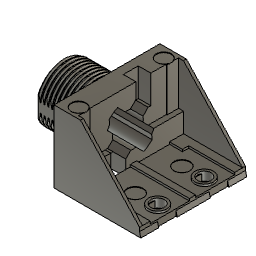
Cherry Pushbutton Base (Autodesk Fusion 360 design; units mm, degrees)
Autodesk Fusion 360 part; units mm, degrees
sketch "Sketch1" plane through (0, 0, 0) normal (0, 1, 0) x (1, 0, 0)
  line L0 (0, 0) -> (0, -14.6844)
  line L1 (0, -14.6844) -> (5.4102, -14.6844)
  line L2 (5.4102, -14.6844) -> (17.4625, -1.778)
  line L3 (17.4625, -1.778) -> (17.4625, 0)
  line L4 (17.4625, 0) -> (0, 0)
  dimension "d12" = 1.778
  dimension "d14" = 17.4625
  dimension "d16" = 14.6844
  dimension "d18" = 5.4102
  constraint coincident L0.start L4.end
  constraint vertical L0
  constraint perpendicular L0 L1
  constraint perpendicular L1 L3
  constraint perpendicular L0 L4
  measures "d12" distance of L2.end L3.end
  measures "d14" distance of L3.end L0.start
  measures "d16" distance of L0.start L0.end
  measures "d18" distance of L0.end L1.end
extrude "Extrude1" add sketch "Sketch1" along normal mid plane 21.6154
ref_plane "WorkPlane1" through (17.4625, 0, 1.778) normal (0, 0, 1) x (0, 1, 0)
sketch "Sketch3" plane through (0, 0, 1.778) normal (0, 0, 1) x (1, 0, 0)
  line L0 (5.4102, -10.8077) -> (5.4102, 10.8077)
  line L1 (17.4625, -10.8077) -> (17.4625, 10.8077)
  line L2 (17.4625, 10.2124) -> (5.4102, 10.2124)
  line L3 (5.4102, 10.2124) -> (5.4102, -10.2124)
  line L4 (5.4102, -10.2124) -> (17.4625, -10.2124)
  line L5 (17.4625, -10.2124) -> (17.4625, 10.2124)
  line L6 (0, 0) -> (5.4102, 0) construction
  dimension "d7" = 20.4248
  constraint horizontal L2
  constraint vertical L3
  constraint horizontal L4
  constraint vertical L5
  constraint coincident L0 L3.end
  constraint coincident L1 L2.start
  constraint coincident L6.start origin
  constraint midpoint L3 L6.end
  constraint horizontal L6
  measures "d7" distance of L2.start L4.end
extrude "Extrude2" cut sketch "Sketch3" along normal up to surface (12.9064 mm away)
sketch "Sketch4" plane through (0, 0, 0) normal (-1, 0, 0) x (0, -1, 0)
  line L0 (10.8077, 14.6844) -> (-10.8077, 14.6844)
  line L1 (-10.8077, 14.6844) -> (-10.8077, 0)
  line L2 (-10.8077, 0) -> (10.8077, 0)
  line L3 (10.8077, 0) -> (10.8077, 14.6844)
  line L4 (-10.8077, 0) -> (10.8077, 14.6844) construction
  circle A0 centre (0, 7.3422) radius 5.3975
  line L5 (-5.3975, 14.6844) -> (5.3975, 14.6844)
  line L6 (5.3975, 14.6844) -> (5.3975, 0)
  line L7 (5.3975, 0) -> (-5.3975, 0)
  line L8 (-5.3975, 0) -> (-5.3975, 14.6844)
  point P0 (0, 7.3422)
  dimension "d87" = 10.795
  constraint coincident L1.end L2.start
  constraint coincident L0.start L3.end
  constraint midpoint L4 P0
  constraint coincident P0 A0.centre
  constraint horizontal L5
  constraint vertical L6
  constraint horizontal L7
  constraint vertical L8
  constraint coincident L2 L6.end
  constraint coincident L0 L5.start
  constraint tangent A0 L6
  constraint tangent A0 L8
  measures "d87" diameter of A0
extrude "Extrude3" add sketch "Sketch4" along normal blind 9.1281 contours A0
sketch "Sketch5" plane through (-9.1281, 0, 0) normal (-1, 0, 0) x (0, -1, 0)
  circle A0 centre (0, 7.3422) radius 4.4323
  circle A1 centre (0, 7.3422) radius 5.3975
  dimension "d33" = 8.8646
  constraint concentric A0 A1
  measures "d33" diameter of A0
extrude "Extrude4" cut sketch "Sketch5" against normal up to surface (14.5383 mm away) contours A0
thread "Thread2" "Custom ANSI Unified Screw Threads 15/32 15/32-32 UN 2A" major diameter 11.684 minor diameter 10.9626 pitch 0.7937 angle 60 modelled right hand crest width 0.2004 on face at (-3.0427, -5.3707, 6.8048) crest through (0.1984, -5.842, 7.3422)
sketch "Sketch6" plane through (5.4102, 0, 0) normal (1, 0, 0) x (0, 1, 0)
  circle A0 centre (0, 7.3422) radius 4.4323
  line L0 (10.2124, 14.6844) -> (-10.2124, 14.6844)
  line L1 (-10.2124, 14.6844) -> (-10.2124, 1.778)
  line L2 (-10.2124, 1.778) -> (10.2124, 1.778)
  line L3 (10.2124, 1.778) -> (10.2124, 14.6844)
  circle A1 centre (0, 7.3422) radius 3.1369
  line L4 (-0.5334, 10.4334) -> (0.5334, 10.4334) construction
  line L5 (0, 14.6844) -> (0, 1.778) construction
  line L6 (0, 10.4791) -> (0, 10.4334) construction
  line L7 (0.5334, 10.4334) -> (1.5824, 11.4824)
  line L8 (-0.5334, 10.4334) -> (-1.5824, 11.4824)
  line L9 (-3.0912, 6.8088) -> (-4.1402, 5.7598)
  line L10 (-3.0912, 6.8088) -> (-3.0912, 7.8756) construction
  line L11 (-3.0912, 7.8756) -> (-4.1402, 8.9246)
  line L12 (-3.1369, 7.3422) -> (-3.0912, 7.3422) construction
  line L13 (0.5334, 4.251) -> (1.5824, 3.202)
  line L14 (0.5334, 4.251) -> (-0.5334, 4.251) construction
  line L15 (-0.5334, 4.251) -> (-1.5824, 3.202)
  line L16 (0, 4.2053) -> (0, 4.251) construction
  line L17 (3.0912, 7.8756) -> (4.1402, 8.9246)
  line L18 (3.0912, 7.8756) -> (3.0912, 6.8088) construction
  line L19 (3.0912, 6.8088) -> (4.1402, 5.7598)
  line L20 (3.1369, 7.3422) -> (3.0912, 7.3422) construction
  line L21 (1.5824, 11.4824) -> (0, 10.4334) construction
  line L22 (-1.5824, 11.4824) -> (0, 10.4334) construction
  line L23 (-4.1402, 5.7598) -> (-4.1402, 0)
  line L24 (-1.5824, 3.202) -> (-1.5824, 0)
  line L25 (10.8077, 0) -> (-10.8077, 0)
  line L26 (-10.2124, 14.6844) -> (10.2124, 14.6844)
  line L27 (10.2124, 14.6844) -> (10.2124, 5.769)
  line L28 (10.2124, 5.769) -> (-10.2124, 5.769)
  line L29 (-10.2124, 5.769) -> (-10.2124, 14.6844)
  circle A2 centre (0, 7.3422) radius 5.0927
  line L30 (-1.5824, 11.4824) -> (-2.0874, 11.9874)
  line L31 (1.5824, 3.202) -> (2.0874, 2.6969)
  line L32 (-2.0874, 11.9874) -> (-3.7985, 10.7343) construction
  line L33 (-3.7985, 10.7343) -> (-3.7214, 9.7497)
  line L34 (-3.6157, 8.4001) -> (-3.7214, 9.7497)
  line L35 (1.5824, 3.202) -> (2.0874, 2.6969)
  line L36 (2.0874, 2.6969) -> (3.7985, 3.95) construction
  line L37 (3.7985, 3.95) -> (3.7214, 4.9346)
  line L38 (3.6157, 6.2843) -> (3.7214, 4.9346)
  point P0 (4.4323, 7.3422)
  point P1 (0, 7.3422)
  point P2 (0, 10.4791)
  point P3 (0, 10.4334)
  point P4 (-3.0912, 7.3422)
  point P5 (-3.1369, 7.3422)
  point P6 (0, 4.251)
  point P7 (0, 4.2053)
  point P8 (3.0912, 7.3422)
  point P9 (3.1369, 7.3422)
  dimension "d38" = 6.2738
  dimension "d39" = 1.0668
  dimension "d41" = 360
  dimension "d72" = 8.9154
  dimension "d88" = 20.4248
  dimension "d90" = 10.1854
  dimension "d92" = 2.1209
  dimension "d94" = 360
  constraint coincident P1 A0.centre
  constraint perpendicular L3 L4
  constraint coincident L5 P2
  constraint coincident A1 P2
  constraint midpoint L4 P3
  constraint coincident P2 L6.start
  constraint coincident P3 L6.end
  constraint vertical L6
  constraint coincident A1 L4.end
  constraint coincident A0 L7.end
  constraint coincident A0 L8.end
  constraint equal L21 L22
  constraint parallel L8 L11
  constraint perpendicular L2 L23
  constraint perpendicular L2 L24
  constraint coincident L23.end L25
  constraint coincident L24.end L25
  constraint horizontal L26
  constraint vertical L27
  constraint horizontal L28
  constraint vertical L29
  constraint coincident L0.end L1.start
  constraint coincident A2 L30.end
  constraint collinear L8 L30
  constraint coincident A2 L31.end
  constraint collinear L13 L31
  constraint coincident A2 L32.end
  constraint coincident A0 L33.end
  constraint coincident L11 L34.start
  constraint midpoint L11 L34.start
  constraint collinear L33 L34
  measures "d38" diameter of A1
  measures "d39" distance of L4.start L4.end
  measures "d72" distance of L0.end L28.end
  measures "d88" distance of L27.end L28.end
  measures "d90" diameter of A2
  measures "d92" distance of L30.end L32.end
extrude "Extrude5" add sketch "Sketch6" against normal blind 7.366 contours A0 A1 L17 L19 L28 | A0 L19 L28 | A0 A1 L7 L8 | A0 A1 L13 L15 | A0 A1 L9 L11 L28 | A0 L9 L28
sketch "Sketch7" plane through (0, 0, 14.6844) normal (0, 0, 1) x (-1, 0, 0)
  line L0 (-5.4102, 10.8077) -> (-5.4102, 10.2124)
  line L1 (-5.4102, 10.2124) -> (-5.4102, -10.2124)
  line L2 (-5.4102, -10.2124) -> (-5.4102, -10.8077)
  line L3 (-5.4102, -10.8077) -> (0, -10.8077)
  line L4 (0, -10.8077) -> (0, 10.8077)
  line L5 (0, 10.8077) -> (-5.4102, 10.8077)
  line L6 (-5.4102, -1.6383) -> (-1.7018, -1.6383)
  line L7 (-1.7018, -1.6383) -> (-1.7018, -4.6863)
  line L8 (-1.7018, -4.6863) -> (-5.4102, -4.6863)
  line L9 (-5.4102, -4.6863) -> (-5.4102, -1.6383)
  line L10 (-3.556, -4.6863) -> (-3.556, -10.8077) construction
  dimension "d50" = 15.494
  dimension "d51" = 12.446
  dimension "d61" = 3.048
  dimension "d62" = 1.7018
  dimension "d64" = 6.1214
  constraint horizontal L6
  constraint vertical L7
  constraint horizontal L8
  constraint vertical L9
  constraint coincident L1 L6.start
  constraint midpoint L8 L10.start
  constraint coincident L3 L10.end
  constraint perpendicular L3 L10
  measures "d50" distance of L5 L8
  measures "d51" distance of L5 L6
  measures "d61" distance of L6.end L7.end
  measures "d62" distance of L4 L7
  measures "d64" distance of L10.start L10.end
extrude "Extrude6" cut sketch "Sketch7" against normal up to surface (5.7598 mm away) contours L1 L6 L7 L8 L9
extrude "Extrude7" cut sketch "Sketch6" against normal up to surface (3.7084 mm away) contours A0 L23 L24 A2 | L2 L23 L24 L25 | L2 L23 L24 A2
sketch "Sketch10" plane through (0, 0, 0) normal (0, 0, -1) x (1, 0, 0)
  line L0 (5.4102, 4.1402) -> (5.4102, 1.5824)
  line L1 (5.4102, 1.5824) -> (1.7018, 1.5824)
  line L2 (1.7018, 1.5824) -> (1.7018, 4.1402)
  line L3 (0, 10.8077) -> (0, -10.8077)
  line L4 (0, -10.8077) -> (17.4625, -10.8077)
  line L5 (17.4625, -10.8077) -> (17.4625, 10.8077)
  line L6 (17.4625, 10.8077) -> (0, 10.8077)
  line L7 (1.7018, 4.1402) -> (5.4102, 4.1402)
sketch "Sketch11" plane through (0, 0, 0) normal (0, 0, -1) x (1, 0, 0)
  line L0 (5.4102, 1.5824) -> (1.7018, 1.5824)
  line L1 (1.7018, 1.5824) -> (1.7018, 4.6304)
  line L2 (1.7018, 4.6304) -> (5.4102, 4.6304)
  line L3 (5.4102, 4.6304) -> (5.4102, 1.5824)
  point P0 (5.4102, 1.5824)
  point P1 (1.7018, 1.5824)
  dimension "d66" = 3.048
  constraint horizontal L0
  constraint vertical L1
  constraint horizontal L2
  constraint vertical L3
  constraint coincident P0 L0.start
  constraint coincident P1 L1
  measures "d66" distance of P0 L2.end
extrude "Extrude9" cut sketch "Sketch11" against normal up to surface (1.778 mm away)
extrude "Extrude10" cut 1 faces at (2.9379, -4.1402, 4.4325) along direction (0, -1, 0) up to surface (0.4902 mm away)
sketch "Sketch12" plane through (0, -4.95, 4.95) normal (0, 0.707107, -0.707107) x (-1, 0, 0)
  line L0 (-5.4102, 2.6287) -> (-5.4102, 1.1452)
  line L1 (-5.4102, 1.1452) -> (-1.7018, 1.1452)
  line L2 (-1.7018, 1.1452) -> (1.9558, 1.1452)
  line L3 (1.9558, 1.1452) -> (1.9558, 2.6287)
  line L4 (1.9558, 2.6287) -> (-5.4102, 2.6287)
extrude "Extrude11" cut sketch "Sketch6" against normal blind 1.143 contours A0 A1 L17 L19 L28 | A0 L28 A2 L30 | A0 L19 L28 | A0 A1 L7 L8 | L0 L1 L3 L26 L27 L28 L29 A2 | A0 A2 L30 L33 | A0 L28 A2 L33 | A0 A1 L9 L11 L28 | A0 L9 L28
sketch "Sketch13" plane through (4.2672, 0, 0) normal (1, 0, 0) x (0, 1, 0)
  line L0 (1.6383, 11.4606) -> (1.6383, 14.6844)
  line L1 (1.6383, 14.6844) -> (-10.2124, 14.6844)
  line L2 (-10.2124, 14.6844) -> (-10.2124, 5.769)
  line L3 (-10.2124, 5.769) -> (-4.1437, 5.769)
  line L4 (-4.1402, 5.7598) -> (-3.0912, 6.8088)
  arc A0 (-3.0912, 7.8756) -> (-3.0912, 6.8088) centre (0, 7.3422) ccw
  line L5 (-3.0912, 7.8756) -> (-4.1402, 8.9246)
  arc A1 (-1.5824, 11.4824) -> (-4.1402, 8.9246) centre (0, 7.3422) ccw
  line L6 (-1.5824, 11.4824) -> (-0.5334, 10.4334)
  arc A2 (0.5334, 10.4334) -> (-0.5334, 10.4334) centre (0, 7.3422) ccw
  line L7 (0.5334, 10.4334) -> (1.5824, 11.4824)
  line L8 (-10.2124, 14.6844) -> (-7.874, 14.6844)
  line L9 (-7.874, 14.6844) -> (-7.874, 5.769)
  line L10 (-7.874, 5.769) -> (-10.2124, 5.769)
  line L11 (-10.2124, 5.769) -> (-10.2124, 14.6844)
  line L12 (10.2124, 5.769) -> (-10.2124, 5.769)
  line L13 (10.2124, 14.6844) -> (10.2124, 5.769)
  line L14 (10.2124, 14.6844) -> (7.874, 14.6844)
  line L15 (7.874, 14.6844) -> (7.874, 5.769)
  line L16 (7.874, 5.769) -> (10.2124, 5.769)
  line L17 (10.2124, 5.769) -> (10.2124, 14.6844)
  arc A3 (-4.1437, 5.769) -> (-4.1402, 5.7598) centre (0, 7.3422) ccw
  arc A4 (1.6383, 11.4606) -> (1.5824, 11.4824) centre (0, 7.3422) ccw
  dimension "d76" = 2.3384
  dimension "d77" = 2.3384
  constraint horizontal L8
  constraint vertical L9
  constraint horizontal L10
  constraint vertical L11
  constraint coincident L1.end L2.start
  constraint collinear L10 L12
  constraint horizontal L14
  constraint vertical L15
  constraint horizontal L16
  constraint vertical L17
  constraint coincident L13.start L14.start
  constraint coincident L9.end L12
  constraint collinear L12 L16
  measures "d76" distance of L1.end L8.end
  measures "d77" distance of L13.start L14.end
extrude "Extrude12" add sketch "Sketch13" along normal blind 0.127 contours L1 L2 L3 L8 L9 L10 L11 L12 | L12 L13 L14 L15 L16 L17
sketch "Sketch14" plane through (0, 0, 14.6844) normal (0, 0, 1) x (-1, 0, 0)
  line L0 (-4.2672, 7.874) -> (-4.2672, -1.6383)
  line L1 (-4.2672, -1.6383) -> (-1.7018, -1.6383)
  line L2 (-1.7018, -1.6383) -> (-1.7018, -4.6863)
  line L3 (-1.7018, -4.6863) -> (-4.2672, -4.6863)
  line L4 (-4.2672, -4.6863) -> (-4.2672, -7.874)
  line L5 (-4.3942, -7.874) -> (-4.3942, -10.2124)
  line L6 (-4.3942, -10.2124) -> (-5.4102, -10.2124)
  line L7 (-5.4102, -10.2124) -> (-5.4102, -10.8077)
  line L8 (-5.4102, -10.8077) -> (0, -10.8077)
  line L9 (0, -10.8077) -> (0, 10.8077)
  line L10 (0, 10.8077) -> (-5.4102, 10.8077)
  line L11 (-5.4102, 10.8077) -> (-5.4102, 10.2124)
  line L12 (-5.4102, 10.2124) -> (-4.3942, 10.2124)
  circle A0 centre (-2.9121, 8.6884) radius 1.524
  circle A1 centre (-2.9121, -8.6884) radius 1.524
  line L13 (-4.2672, -7.874) -> (-4.3942, -7.874)
  line L14 (-4.3942, 10.2124) -> (-4.3942, 7.874)
  line L15 (-4.3942, 7.874) -> (-4.2672, 7.874)
  point P0 (-4.3942, 9.0432)
  point P1 (-4.3942, -9.0432)
  dimension "d83" = 3.048
  constraint equal A0 A1
  constraint coincident A0 P0
  constraint midpoint P0 L14
  constraint coincident A1 P1
  constraint midpoint L5 P1
  constraint tangent L12 A0
  constraint tangent L6 A1
  measures "d83" diameter of A0
extrude "Extrude13" cut sketch "Sketch14" against normal blind 0.127 contours A0 L14 | L5 A1 picked at (-3.376, 8.2464) picked at (-3.7379, -8.9714)
extrude "Extrude14" cut sketch "Sketch6" against normal up to surface (14.5383 mm away) contours A0 A2 L30 L33 | A0 A2 L31 L35 L37
sketch "Sketch15" plane through (-9.1281, 0, 0) normal (-1, 0, 0) x (0, -1, 0)
  line L0 (-1.5824, 3.202) -> (-2.0874, 2.6969)
  arc A0 (-3.7985, 3.95) -> (-2.0874, 2.6969) centre (0, 7.3422) ccw
  line L1 (-3.7985, 3.95) -> (-3.7214, 4.9346)
  line L2 (1.5824, 11.4824) -> (2.0874, 11.9874)
  arc A1 (3.7985, 10.7343) -> (2.0874, 11.9874) centre (0, 7.3422) ccw
  line L3 (3.7985, 10.7343) -> (3.7214, 9.7497)
  circle A2 centre (0, 7.3422) radius 5.0927
  arc A3 (-1.5824, 3.202) -> (3.7214, 9.7497) centre (0, 7.3422) ccw
  arc A4 (1.5824, 11.4824) -> (-3.7214, 4.9346) centre (0, 7.3422) ccw
  spline S0 degree 3 poles (-3.5319, 11.5339) (-4.0995, 11.0932) (-4.5748, 10.5451) (-5.2959, 9.2888) (-5.5312, 8.5907) (-5.7243, 7.1327) (-5.6762, 6.3863) (-5.3692, 5.2213) (-5.197, 4.7889) (-4.7511, 3.9707) (-4.4781, 3.5885) (-4.1624, 3.243) knots 0 0 0 0 0.215586 0.215586 0.434425 0.434425 0.656519 0.656519 0.795513 0.795513 0.935766 0.935766 0.935766 0.935766
  arc A5 (-4.1624, 3.243) -> (4.1624, 3.243) centre (0, 7.3422) ccw
  spline S1 degree 3 poles (4.1624, 3.243) (4.6715, 3.8002) (5.0677, 4.4508) (5.5827, 5.8578) (5.7005, 6.5991) (5.6436, 8.0741) (5.4737, 8.7937) (4.9841, 9.8671) (4.7501, 10.2504) (4.1976, 10.9489) (3.8819, 11.2621) (3.5319, 11.5339) knots 0 0 0 0 0.226441 0.226441 0.449625 0.449625 0.669553 0.669553 0.803905 0.803905 0.936997 0.936997 0.936997 0.936997
  arc A6 (3.5319, 11.5339) -> (-3.5319, 11.5339) centre (0, 7.3422) ccw
  circle A7 centre (0, 7.3422) radius 10.8077
  dimension "d104" = 21.6154
  constraint concentric A2 A7
  measures "d104" diameter of A7
extrude "Extrude16" cut sketch "Sketch15" against normal blind 0.508 contours S0 A5 S1 A6 | A7
fillet "Fillet3" radius 0.254 2 edges at (-9.1281, -4.1088, 4.3332) (-9.1281, 4.1088, 10.3511)
extrude "Extrude17" cut sketch "Sketch4" along normal up to surface (8.6201 mm away) contours L0 L2 L3 L6 | L0 L1 L2 L8
sketch "Sketch16" plane through (0, 0, 1.778) normal (0, 0, 1) x (-1, 0, 0)
  line L0 (-17.4625, 10.2124) -> (-17.4625, -10.2124)
  line L1 (-17.4625, -10.2124) -> (-5.4102, -10.2124)
  line L2 (-5.4102, -10.2124) -> (-5.4102, 1.5824)
  line L3 (-5.4102, 1.5824) -> (-5.4102, 4.6304)
  line L4 (-5.4102, 4.6304) -> (-5.4102, 10.2124)
  line L5 (-5.4102, 10.2124) -> (-17.4625, 10.2124)
  line L6 (-17.4625, 8.6169) -> (-8.0645, 8.617)
  line L7 (-8.0645, 8.617) -> (-8.0645, 7.3533)
  line L8 (-8.0645, 7.3533) -> (-5.4102, 7.3533)
  line L9 (-5.4102, -7.3533) -> (-8.0645, -7.3533)
  line L10 (-8.0645, -7.3533) -> (-8.0645, -8.6169)
  line L11 (-8.0645, -8.6169) -> (-17.4625, -8.617)
  line L12 (-17.4625, -0.635) -> (-5.4102, -0.635)
  line L13 (-17.4625, 0.635) -> (-5.4102, 0.635)
  line L14 (0, 0) -> (-17.4625, 0) construction
  line L15 (-11.4363, -0.635) -> (-11.4363, 0.635) construction
  line L16 (-12.7635, 8.6169) -> (-12.7635, -8.6169) construction
  line L17 (-5.4102, 7.3533) -> (-5.4102, -7.3533) construction
  circle A0 centre (-15.1003, 4.7625) radius 1.3843
  circle A1 centre (-15.1003, -4.7625) radius 1.3843
  line L18 (-15.1003, 4.7625) -> (-15.1003, -4.7625) construction
  line L19 (-13.8938, -6.1468) -> (-16.3068, -6.1468) construction
  line L20 (-16.3068, -6.1468) -> (-16.3068, 6.1468)
  line L21 (-16.3068, 6.1468) -> (-13.8938, 6.1468) construction
  line L22 (-13.8938, 6.1468) -> (-13.8938, -6.1468)
  line L23 (-13.8938, -6.1468) -> (-16.3068, 6.1468) construction
  line L24 (-16.3068, -6.1468) -> (-13.8938, 6.1468) construction
  circle A2 centre (-15.1003, 4.7625) radius 1.8923
  circle A3 centre (-15.1003, -4.7625) radius 1.8923
  circle A4 centre (-10.5283, 4.7625) radius 1.6383
  circle A5 centre (-10.5283, -4.7625) radius 1.6383
  line L25 (-15.1003, 4.7625) -> (-10.5283, 4.7625) construction
  line L26 (-10.5283, 4.7625) -> (-10.5283, -4.7625) construction
  line L27 (-10.5283, -4.7625) -> (-15.1003, -4.7625) construction
  point P0 (-11.4363, 0)
  point P1 (-12.7635, 0)
  point P2 (-15.1003, 0)
  point P3 (-15.1003, 0)
  dimension "d112" = 1.27
  dimension "d113" = 17.2339
  dimension "d114" = 9.398
  dimension "d115" = 14.7066
  dimension "d116" = 2.7686
  dimension "d118" = 9.525
  dimension "d119" = 2.3622
  dimension "d120" = 2.413
  dimension "d121" = 3.7846
  dimension "d122" = 3.2766
  dimension "d123" = 4.572
  dimension "d130" = 7.9819
  constraint coincident L0 L6.start
  constraint perpendicular L4 L6
  constraint perpendicular L6 L7
  constraint coincident L4 L8.end
  constraint perpendicular L4 L8
  constraint coincident L2 L9.start
  constraint perpendicular L2 L9
  constraint perpendicular L9 L10
  constraint coincident L0 L11.end
  constraint perpendicular L0 L11
  constraint coincident L0 L12.start
  constraint coincident L2 L12.end
  constraint perpendicular L2 L12
  constraint coincident L0 L13.start
  constraint coincident L2 L13.end
  constraint perpendicular L2 L13
  constraint collinear L7 L10
  constraint equal L7 L10
  constraint coincident L14.start origin
  constraint midpoint L0 L14.end
  constraint midpoint L12 L15.start
  constraint midpoint L13 L15.end
  constraint midpoint L15 P0
  constraint coincident L14 P0
  constraint midpoint L6 L16.start
  constraint midpoint L11 L16.end
  constraint midpoint L16 P1
  constraint coincident L14 P1
  constraint equal A0 A1
  constraint coincident A0.centre L18.start
  constraint coincident A1.centre L18.end
  constraint vertical L18
  constraint midpoint L18 P3
  constraint coincident L14 P3
  constraint horizontal L19
  constraint perpendicular L19 L20
  constraint parallel L19 L21
  constraint parallel L20 L22
  constraint coincident L23 P3
  constraint coincident L24 P3
  constraint coincident P3 P2
  constraint concentric A1 A3
  constraint equal A2 A3
  constraint equal A4 A5
  constraint coincident A4.centre L25.end
  constraint perpendicular L16 L25
  constraint coincident A5.centre L26.end
  constraint perpendicular L12 L26
  constraint perpendicular L18 L27
  constraint tangent A0 L21
  measures "d112" distance of L12 L13
  measures "d113" distance of L16.start L16.end
  measures "d114" distance of L10.end L11.end
  measures "d115" distance of L8.end L9.start
  measures "d116" diameter of A0
  measures "d118" distance of A0.centre A1.centre
  measures "d119" distance of L0 L18
  measures "d120" distance of L20.end L21.end
  measures "d121" diameter of A2
  measures "d122" diameter of A4
  measures "d123" distance of A0.centre A4.centre
  measures "d130" distance of L6 L13
extrude "Extrude18" cut sketch "Sketch16" against normal blind 1.778 contours A0 L20 L22 | A1 L20 L22
extrude "Extrude19" cut sketch "Sketch16" against normal blind 0.4318 contours L0 L2 L3 L4 L6 L7 L8 L13 L20 L22 A2 | L0 L2 L9 L10 L11 L12 L20 L22 A3 | L13 L20 L22 A2 | L12 L20 L22 A3 | A0 L20 | A1 L20 | A0 L22 | A1 L22
extrude "Extrude20" cut sketch "Sketch16" against normal blind 0.5588 contours A4 | A5
sketch "Sketch17" plane through (17.4625, 0, 0) normal (1, 0, 0) x (0, 1, 0)
  line L0 (-8.6169, 1.3462) -> (-8.6169, 1.778)
  line L1 (-8.6169, 1.778) -> (-10.2124, 1.778)
  line L2 (-10.2124, 1.778) -> (-10.8077, 1.778)
  line L3 (-10.8077, 1.778) -> (-10.8077, 0)
  line L4 (-10.8077, 0) -> (10.8077, 0)
  line L5 (10.8077, 0) -> (10.8077, 1.778)
  line L6 (10.8077, 1.778) -> (10.2124, 1.778)
  line L7 (10.2124, 1.778) -> (8.617, 1.778)
  line L8 (8.617, 1.778) -> (8.617, 1.3462)
  line L9 (8.617, 1.3462) -> (0.635, 1.3462)
  line L10 (0.635, 1.3462) -> (0.635, 1.778)
  line L11 (0.635, 1.778) -> (-0.635, 1.778)
  line L12 (-0.635, 1.778) -> (-0.635, 1.3462)
  line L13 (-0.635, 1.3462) -> (-8.6169, 1.3462)
  line L14 (10.8077, 0) -> (7.1628, 0)
  line L15 (7.1628, 0) -> (7.1628, 1.016)
  line L16 (7.1628, 1.016) -> (10.8077, 1.016)
  line L17 (10.8077, 1.016) -> (10.8077, 0)
  line L18 (-10.8077, 0) -> (-7.1628, 0)
  line L19 (-7.1628, 0) -> (-7.1628, 1.016)
  line L20 (-7.1628, 1.016) -> (-10.8077, 1.016)
  line L21 (-10.8077, 1.016) -> (-10.8077, 0)
  line L22 (-3.3731, 0) -> (3.3731, 0)
  line L23 (3.3731, 0) -> (3.3731, 1.016)
  line L24 (3.3731, 1.016) -> (-3.3731, 1.016)
  line L25 (-3.3731, 1.016) -> (-3.3731, 0)
  dimension "d131" = 3.6449
  dimension "d132" = 1.016
  dimension "d133" = 6.7462
  constraint horizontal L14
  constraint vertical L15
  constraint horizontal L16
  constraint vertical L17
  constraint coincident L4.end L5.start
  constraint horizontal L18
  constraint vertical L19
  constraint horizontal L20
  constraint vertical L21
  constraint coincident L3.end L4.start
  constraint equal L15 L19
  constraint equal L16 L20
  constraint horizontal L22
  constraint vertical L23
  constraint horizontal L24
  constraint vertical L25
  constraint equal L15 L23
  constraint midpoint L22 origin
  measures "d131" distance of L4.end L14.end
  measures "d132" distance of L4.end L16.end
  measures "d133" distance of L22.start L22.end
extrude "Extrude22" add sketch "Sketch17" along normal blind 0.254 contours L3 L4 L18 L19 L20 L21 | L4 L22 L23 L24 L25 | L4 L5 L14 L15 L16 L17
sketch "Sketch19" plane through (0, -3.3731, 0) normal (0, -1, 0) x (1, 0, 0)
  line L0 (17.4625, 1.016) -> (17.4625, 0)
  line L1 (17.7165, 0) -> (17.7165, 1.016)
  line L2 (17.7165, 1.016) -> (17.4625, 1.016)
  line L3 (17.4625, 1.016) -> (17.7165, 1.016)
  line L4 (17.7165, 0) -> (17.7165, 1.016)
  line L5 (17.4625, 1.016) -> (17.7165, 0)
  constraint coincident L0.start L2.end
  constraint coincident L1.end L2.start
  constraint coincident L1.start L4.start
extrude "Extrude23" cut sketch "Sketch19" along normal up to surface (7.4346 mm away) and the other way up to surface (14.1808 mm away)
equation "d1 = OutsideLength"
equation "d7 = InsideLength"
equation "d12 = BaseThickness"
equation "d14 = Width"
equation "d16 = Height"
equation "d18 = FullTopDepth"
equation "d19 = ThreadLength"
equation "OutsideLength = 0.851 in"
equation "InsideLength = OutsideLength - ( 2 * SideThickness )"
equation "BaseThickness = 0.07 in"
equation "SideThickness = ( 3 / 128 ) * 1 in"
equation "Width = ( 11 / 16 ) * 1 in"
equation "Height = ( 37 / 64 ) * 1 in"
equation "TopLipDistance = 0.168 in"
equation "ThreadLength = ( 23 / 64 ) * 1 in"
equation "d33 = InsideDiameter"
equation "InsideDiameter = 0.349 in"
equation "FrontThickness = 0.177 in"
equation "d38 = InnerTriangleDiameter"
equation "d39 = InnerTrianglePlateu"
equation "d42 = -( 0.53 in - 0.24 in )"
equation "d51 = LongTopReliefDistance"
equation "InnerTriangleDiameter = 0.247 in"
equation "InnerTrianglePlateu = 0.042 in"
equation "ShortLegReliefWidth = 0.120 in"
equation "d61 = ShortLegReliefWidth"
equation "d62 = ShortLegReliefFromFront"
equation "ShortLegReliefFromFront = 0.067 in"
equation "LongTopReliefDistance = 0.490 in"
equation "d66 = ShortLegReliefWidth"
equation "FullTopDepth = 0.213 in"
equation "d73 = -( FullTopDepth - TopLipDistance )"
equation "SideFeatureWidth = 0.1155 in - SideThickness"
equation "d76 = SideFeatureWidth"
equation "d77 = SideFeatureWidth"
equation "d78 = Bump"
equation "Bump = 0.005 in"
equation "CircleFeatureDiameter = 0.12 in"
equation "d83 = CircleFeatureDiameter"
equation "d84 = -Bump"
equation "ThreadSize = 0.425 in"
equation "d87 = ThreadSize"
equation "d88 = InsideLength"
equation "LongLegExtraDiameter = 0.401 in"
equation "d90 = LongLegExtraDiameter"
equation "ExtraLength = 0.0835 in"
equation "d92 = ExtraLength"
equation "d104 = OutsideLength"
equation "d105 = -ThreadLip"
equation "d108 = 2 * Bump"
equation "ThreadLip = 0.020 in"
equation "d128 = -1 * ( 0.017 in + Bump )"
